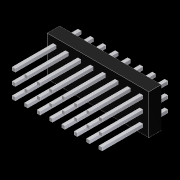
# Autodesk Inventor part: J21
Saved by Autodesk Inventor 2012 (Build 160160000, 160)
## iProperties
Company: Team 801
Created: 2009-08-01
Part Number: J21
Document SubType Name: Modeling
Designer: Jeffrey M
Density: 1 g/cm^3
Catalog Web Link: www.team801.org
Material: Default
Mass: 0.535693 g
Surface Area: 11.5148 cm^2
Volume: 0.535693 cm^3
Author: Jeffrey M
Autodesk Inventor part; units mm, degrees
ref_plane "YZ Plane" through (0, 0, 0) normal (1, 0, 0) x (0, 1, 0)
ref_plane "XZ Plane" through (0, 0, 0) normal (0, 1, 0) x (-1, 0, 0)
ref_plane "XY Plane" through (0, 0, 0) normal (0, 0, 1) x (1, 0, 0)
sketch "Sketch1" plane through (0, 0, 0) normal (0, 0, 1) x (1, 0, 0)
  line L0 (0, 0) -> (20.828, 0)
  line L1 (20.828, -8.128) -> (0, -8.128)
  line L2 (20.828, 0) -> (20.828, -8.128)
  line L3 (0, -8.128) -> (0, 0)
  line L4 (19.6215, -1.8415) -> (19.6215, -1.2065)
  line L5 (19.6215, -1.2065) -> (18.9865, -1.2065)
  line L6 (18.9865, -1.2065) -> (18.9865, -1.8415)
  line L7 (18.9865, -1.8415) -> (19.6215, -1.8415)
  constraints: 16 end point
extrude "Extrusion1" add sketch "Sketch1" against normal blind 2.54
extrude "Extrusion2" add sketch "Sketch1" along normal blind 8.382 contours L7 L6 L5 L4
extrude "Extrusion3" add sketch "Sketch1" against normal blind 5.08 contours L7 L6 L5 L4
pattern_linear "Rectangular Pattern1" count 3 spacing 2.54 along (0, -1, 0) count 8 spacing 2.54 along (-1, 0, 0) of "Extrusion3", "Extrusion2"
body "Solid1"
